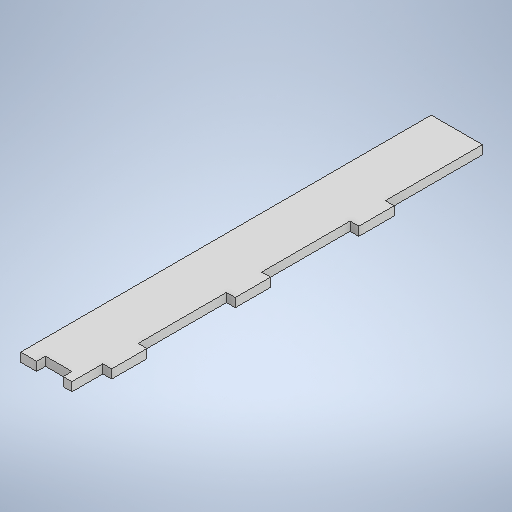
# Autodesk Inventor part: Manija1
Saved by Autodesk Inventor 2025 (Build 290162000, 162)
## iProperties
Created: 2024-11-21
Part Number: Manija1
Material: Generic
Document SubType Name: Sheet Metal
Designer: g.marin
Density: 1 g/cm^3
Sheet Metal Rule: Default
Appearance: Default
Author: g.marin
Autodesk Inventor part; units mm, degrees
ref_plane "YZ Plane" through (0, 0, 0) normal (1, 0, 0) x (0, 1, 0)
ref_plane "XZ Plane" through (0, 0, 0) normal (0, 1, 0) x (-1, 0, 0)
ref_plane "XY Plane" through (0, 0, 0) normal (0, 0, 1) x (1, 0, 0)
sketch "Sketch1" plane through (0, 0, 0) normal (0, 1, 0) x (-1, 0, 0)
  line L0 (-14.5, 116.25) -> (14.5, 116.25)
  line L1 (14.5, 116.25) -> (14.5, -116.25)
  line L2 (14.5, -116.25) -> (-14.5, -116.25)
  line L3 (-14.5, -116.25) -> (-14.5, 116.25)
  line L4 (-14.5, 116.25) -> (14.5, -116.25) construction
  line L5 (14.5, 116.25) -> (-14.5, -116.25) construction
  line L6 (-14.5, 98.75) -> (-19.5, 98.75)
  line L7 (-19.5, 98.75) -> (-19.5, 78.75)
  line L8 (-19.5, 78.75) -> (-14.5, 78.75)
  line L9 (-14.5, 78.75) -> (-14.5, 98.75)
  line L10 (-14.5, 28.75) -> (-19.5, 28.75)
  line L11 (-19.5, 28.75) -> (-19.5, 8.75)
  line L12 (-19.5, 8.75) -> (-14.5, 8.75)
  line L13 (-14.5, 8.75) -> (-14.5, 28.75)
  line L14 (-14.5, -41.25) -> (-19.5, -41.25)
  line L15 (-19.5, -41.25) -> (-19.5, -61.25)
  line L16 (-19.5, -61.25) -> (-14.5, -61.25)
  line L17 (-14.5, -61.25) -> (-14.5, -41.25)
  line L18 (5.5, 116.25) -> (-9.5, 116.25)
  line L19 (-9.5, 116.25) -> (-9.5, 111.25)
  line L20 (-9.5, 111.25) -> (5.5, 111.25)
  line L21 (5.5, 111.25) -> (5.5, 116.25)
  point P0 (0, 0)
  point P1 (-9.5, 116.25)
  dimension "d0" = 29
  dimension "d1" = 232.5
  dimension "d2" = 5
  dimension "d3" = 20
  dimension "d4" = 20
  dimension "d5" = 20
  dimension "d6" = 50
  dimension "d7" = 50
  dimension "d8" = 17.5
  dimension "d9" = 5
  dimension "d10" = 15
  dimension "d11" = 9
  constraints: 44 end point, 10 parallel, 6 point on line, 5 horizontal, 5 perpendicular, 2 midpoint
  measures "d0" distance of L1.end L2.end
  measures "d1" distance of L0.end L1.end
  measures "d2" distance of L6.start L6.end
  measures "d3" distance of L6.end L7.end
  measures "d4" distance of L10.end L11.end
  measures "d5" distance of L14.end L15.end
  measures "d6" distance of L10.end L7.end
  measures "d7" distance of L14.end L11.end
  measures "d8" vertical distance of L0.start L6.end
  measures "d9" distance between parallel lines of L20 L0
  measures "d10" distance of L19.end L20.end
  measures "d11" distance between parallel lines of L1 L21
extrude "Extrusion1" add sketch "Sketch1" along normal blind 5 contours L0 L19 L20 L21 L1 L2 L3 | L3 L8 L7 L6 | L3 L12 L11 L10 | L3 L16 L15 L14
equation "\"BendRadius\" = Thickness"
equation "\"BendReliefWidth\" = Thickness"
equation "\"BendReliefDepth\" = 0.5 * Thickness"
equation "\"CornerReliefSize\" = 4 * Thickness"
equation "\"MinimumRemnant\" = 2 * Thickness"
equation "\"TransitionRadius\" = BendRadius"
equation "\"JacobiRadiusSize\" = BendRadius"
equation "\"GapSize\" = Thickness"
equation "\"Thickness\" = 3.048"
body "Solid1"
